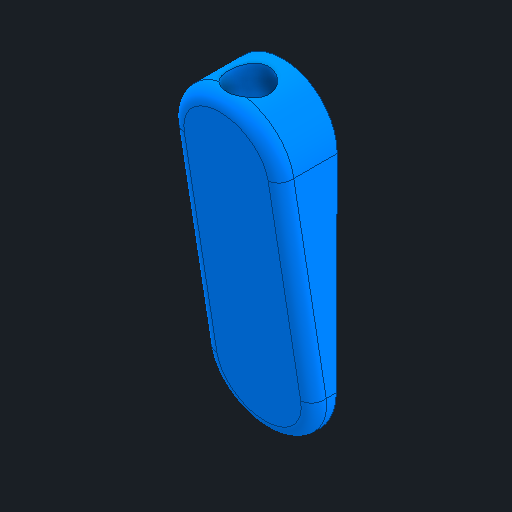
# Autodesk Inventor part: shaft_outlet
Saved by Autodesk Inventor 2022.2 (Build 262287010, 287A)
## iProperties
Created: 2022-03-28
Part Number: shaft_outlet
Material: Generic
Document SubType Name: Modeling
Designer: kardo
Density: 1 g/cm^3
Appearance: Blue Plastic
Author: kardo
Autodesk Inventor part; units mm, degrees
ref_plane "YZ Plane" through (0, 0, 0) normal (1, 0, 0) x (0, 1, 0)
ref_plane "XZ Plane" through (0, 0, 0) normal (0, 1, 0) x (-1, 0, 0)
ref_plane "XY Plane" through (0, 0, 0) normal (0, 0, 1) x (1, 0, 0)
derived "stencil_frame.ipt"
sketch "sk_drivetrain_profile" plane through (6, 0, 0) normal (1, 0, 0) x (0, 1, 0)
  line L0 (-548.1262, 0) -> (397.7572, 0) construction
  line L1 (-363, 1541.8302) -> (-363, -1877.3857) construction
  line L2 (0, 1541.8302) -> (0, -1877.3857) construction
  line L3 (-140.12, 52.421) -> (-133.3462, 25.2528)
  line L4 (-388, 0) -> (-343.0839, 2.7472)
  line L5 (-136.7331, 38.8369) -> (-223.8252, 17.1224)
  line L6 (-300.1691, 5.372) -> (-261.4573, 7.7397) construction
  line L7 (-261.4573, 7.7397) -> (-223.8252, 17.1224) construction
  line L8 (-133.3462, 25.2528) -> (-133.3462, 20.2528) construction
  line L9 (-343.0839, 2.7472) -> (-300.1691, 5.372)
  line L10 (-513.6167, 1550.4344) -> (344.3546, -1890.7004) construction
  spline S0 degree 2 poles (-300.1691, 5.372) (-261.4573, 7.7397) (-223.8252, 17.1224) knots 1 1 1 2 2 2
  line L11 (-224.4013, 19.4329) -> (-137.3092, 41.1474) construction
  line L12 (-136.1571, 36.5264) -> (-223.2491, 14.8119) construction
  line L13 (-224.4013, 19.4329) -> (-223.2491, 14.8119) construction
  line L14 (0, 18.496) -> (-254.1001, 19.5569) construction
  line L15 (-55.187, 19.9264) -> (-309.3336, 20.9876) construction
  point P0 (0, 0)
  point P1 (-214.7203, 19.3925)
  point P2 (-205.0394, 19.3521)
  point P3 (-200.3057, 20.5323)
sketch "sk_prop_shaft_cut" plane through (6, 0, 18.496) normal (0, 0.0041752, 0.9999913) x (0, -0.9999913, 0.0041752)
  line L0 (224.4032, -4.3812) -> (200.3124, -4.3812)
  line L1 (224.4032, 4.3812) -> (200.3124, 4.3812)
  arc A0 (200.3124, 4.3812) -> (200.3124, -4.3812) centre (200.3124, 0) ccw
  arc A1 (224.4032, -4.3812) -> (224.4032, 4.3812) centre (224.4032, 0) ccw
  point P0 (-0.0772, -6)
  point P1 (214.7222, 0)
  point P2 (224.4032, 0)
  point P3 (205.0412, 0)
  point P4 (200.3124, 0)
ref_plane "plane_motor_mount" through (0, -127.05, 0) normal (0, 0.9702957, 0.2419219) x (-1, 0, 0)
derived "parameters_powertrain.ipt"
derived "parameters_frame.ipt"
extrude "lower_plate" add sketch "sk_prop_shaft_cut" along normal blind 1.2
sketch "sk_upper_plate" plane through (6, -224.3962, 20.6329) normal (0, 0.0041752, 0.9999913) x (1, 0, 0)
  line L0 (-4.3812, 24.0908) -> (-4.3812, 0) projected
  arc A0 (-4.3812, 0) -> (4.3812, 0) centre (0, 0) ccw projected
  line L1 (4.3812, 0) -> (4.3812, 24.0908) projected
  arc A1 (4.3812, 24.0908) -> (-4.3812, 24.0908) centre (0, 24.0908) ccw projected
  line L2 (-6.3812, 0) -> (-6.3813, 24.0908)
  arc A2 (6.3812, 24.0908) -> (-6.3813, 24.0908) centre (0, 24.0908) ccw
  line L3 (6.3812, 24.0908) -> (6.3812, 0)
  arc A3 (-6.3812, 0) -> (6.3812, 0) centre (0, 0) ccw
  point P0 (-6, 224.4804)
  dimension "d6" = 2
  constraints: 4 end point, 4 point on circle, 2 centre point, 3 other
  measures "d6" distance between parallel lines of L2 L0
extrude "upper_plate" add sketch "sk_upper_plate" along normal blind 7.62 contours A1 L1 A0 L0 | L2 A2 L3 A3
sketch "sk_trim" plane through (12.3812, -224.3962, 20.6329) normal (1, 0, 0) x (0, -0.0041752, -0.9999913)
  line L0 (-1.6669, -6.3813) -> (-7.62, 30.472)
  line L1 (0, 0) -> (0, -6.3812) projected
  line L2 (-7.62, 30.472) -> (-7.62, 24.0908) projected
  line L3 (0, -6.3812) -> (-1.6669, -6.3813)
  line L4 (-1.6669, -6.3813) -> (-7.62, -6.3813)
  line L5 (-7.62, -6.3813) -> (-7.62, 24.0908)
  dimension "d16" = 1.6669
  constraints: 8 end point, 2 collinear, 1 perpendicular
  measures "d16" distance of L1.end L0.start
extrude "trim" cut sketch "sk_trim" against normal through all
sketch "sk_drill" plane through (0, -127.05, 0) normal (0, 0.9702957, 0.2419219) x (-1, 0, 0)
  circle A0 centre (-6, 40.0258) radius 2.3813
  point P0 (0, -30.7362)
  dimension "d9" = 4.7625
  constraints: 1 centre point, 1 coincident
  measures "d9" diameter of A0
extrude "drill" cut sketch "sk_drill" along normal through all both and the other way through all
fillet "Fillet1" radius 1.5 6 edges at (10.5122, -228.9002, 22.6205) (1.4878, -228.9002, 22.6205) (-0.3812, -212.3316, 25.226) (10.5122, -195.7629, 27.8315) (1.4878, -195.7629, 27.8315) (12.3812, -212.3316, 25.226)
equation "\"d4\" = shell_thickness"
equation "\"d7\" = 1.6 * prop_shaft_od"
equation "\"d16\" = 0.35 * prop_shaft_od"
equation "\"d9\" = prop_shaft_od"
equation "\"shell_thickness\" = 1.2"
equation "\"prop_shaft_od\" = 4.7625"
body "Solid1"
